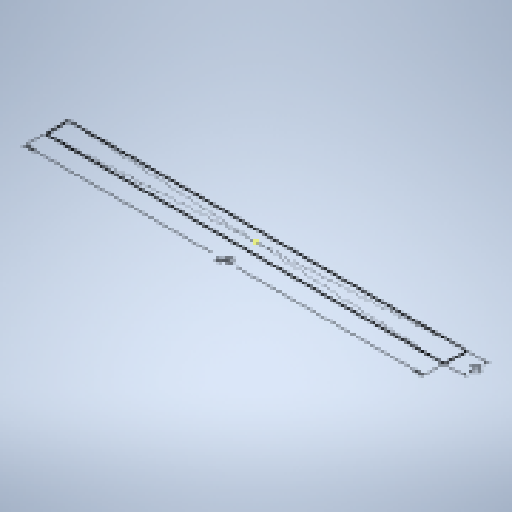
# Autodesk Inventor part: ДМС 053 усилитель кормовой 1
Saved by Autodesk Inventor 2024.2 (Build 282272000, 272)
## iProperties
Created: 2024-05-13
Part Number: ДМС 053 усилитель кормовой 1
Material: Generic
Document SubType Name: Modeling
Designer: admin
Density: 1 g/cm^3
Appearance: Default
Author: admin
Autodesk Inventor part; units mm, degrees
ref_plane "YZ Plane" through (0, 0, 0) normal (1, 0, 0) x (0, 1, 0)
ref_plane "XZ Plane" through (0, 0, 0) normal (0, 1, 0) x (-1, 0, 0)
ref_plane "XY Plane" through (0, 0, 0) normal (0, 0, 1) x (1, 0, 0)
sketch "Sketch1" plane through (0, 0, 0) normal (0, 0, 1) x (1, 0, 0)
  line L0 (-220, 12.5) -> (220, 12.5)
  line L1 (220, 12.5) -> (220, -12.5)
  line L2 (220, -12.5) -> (-220, -12.5)
  line L3 (-220, -12.5) -> (-220, 12.5)
  line L4 (-220, 12.5) -> (220, -12.5) construction
  line L5 (220, 12.5) -> (-220, -12.5) construction
  point P0 (0, 0)
  dimension "d0" = 440
  dimension "d1" = 25
  constraints: 12 end point, 2 midpoint, 2 parallel, 1 horizontal, 1 perpendicular
  measures "d0" distance of L1.end L2.end
  measures "d1" distance of L0.end L1.end
extrude "Extrusion1" add sketch "Sketch1" along normal blind 10
body "Solid1"
